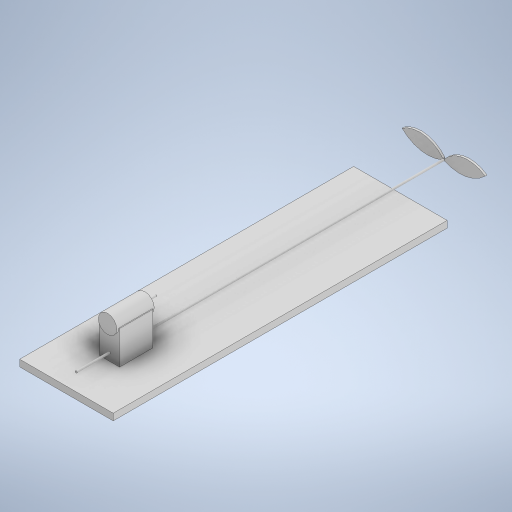
# Autodesk Inventor part: Motor Shaft
Saved by Autodesk Inventor 2024 (Build 280153000, 153)
## iProperties
Created: 2024-09-04
Part Number: Motor Shaft
Material: Generic
Document SubType Name: Modeling
Designer: srira
Density: 1 g/cm^3
Appearance: Default
Author: srira
Autodesk Inventor part; units mm, degrees
ref_plane "YZ Plane" through (0, 0, 0) normal (1, 0, 0) x (0, 1, 0)
ref_plane "XZ Plane" through (0, 0, 0) normal (0, 1, 0) x (-1, 0, 0)
ref_plane "XY Plane" through (0, 0, 0) normal (0, 0, 1) x (1, 0, 0)
sketch "Sketch1" plane through (0, 0, 0) normal (0, 1, 0) x (-1, 0, 0)
  line L0 (-70, 250) -> (70, 250)
  line L1 (70, 250) -> (70, -250)
  line L2 (70, -250) -> (-70, -250)
  line L3 (-70, -250) -> (-70, 250)
  line L4 (-70, 250) -> (70, -250) construction
  line L5 (70, 250) -> (-70, -250) construction
  point P0 (0, 0)
  dimension "d0" = 140
  dimension "d1" = 500
  constraints: 12 end point, 2 midpoint, 2 parallel, 1 horizontal, 1 perpendicular
  measures "d0" distance of L1.end L2.end
  measures "d1" distance of L0.end L1.end
extrude "Extrusion1" add sketch "Sketch1" along normal blind 10
sketch "Sketch2" plane through (0, 10, 0) normal (0, 1, 0) x (1, 0, 0)
  line L0 (15, -185.42) -> (-15, -185.42)
  line L1 (-15, -185.42) -> (-15, -135.42)
  line L2 (-15, -135.42) -> (15, -135.42)
  line L3 (15, -135.42) -> (15, -185.42)
  line L4 (15, -185.42) -> (-15, -135.42) construction
  line L5 (-15, -185.42) -> (15, -135.42) construction
  point P0 (0, 0)
  point P1 (0, -160.42)
  dimension "d4" = 30
  dimension "d5" = 50
  constraints: 12 end point, 2 midpoint, 2 parallel, 1 horizontal, 1 perpendicular
  measures "d4" distance of L1.end L2.end
  measures "d5" distance of L0.end L1.end
extrude "Extrusion2" add sketch "Sketch2" along normal blind 50
sketch "Sketch3" plane through (15, 10, 135.42) normal (0, 0, -1) x (-1, 0, 0)
  line L0 (30, 50) -> (0, 50) projected
  circle A0 centre (15, 50) radius 13.8
  point P0 (15, -10)
  point P1 (1.2, 50)
  point P2 (28.8, 50)
  dimension "d8" = 27.6
  constraints: 1 centre point, 1 midpoint
  measures "d8" diameter of A0
extrude "Extrusion3" cut sketch "Sketch3" against normal blind 50 contours A0 L0 picked at (18.5768, 45.8488)
sketch "Sketch4" plane through (-15, 10, 185.42) normal (0, 0, 1) x (1, 0, 0)
  circle A0 centre (15, 11.2668) radius 1.5
  point P0 (15, -10)
  dimension "d11" = 3
  constraints: 1 centre point
  measures "d11" diameter of A0
extrude "Extrusion5" add sketch "Sketch4" along normal blind 50 and the other way blind 500
sketch "Sketch5" plane through (0, 21.2668, -314.58) normal (0, 0, -1) x (-1, 0, 0)
  circle A0 centre (0, 0) radius 1.5 projected
  arc A1 (62.1392, 9.8676) -> (0, 0) centre (36.1239, -26.8945) ccw
  arc A2 (0, 0) -> (62.1392, 9.8676) centre (24.2766, 47.7112) ccw
  arc A3 (0, 0) -> (-62.1392, 9.8676) centre (-36.1239, -26.8945) ccw
  arc A4 (-62.1392, 9.8676) -> (0, 0) centre (-24.2766, 47.7112) ccw
  point P0 (0, -21.2668)
  point P1 (1.3463, -0.6614)
  point P2 (0.9157, 1.1881)
  point P3 (-1.3463, -0.6614)
  point P4 (-0.9157, 1.1881)
  constraints: 8 point on circle, 4 centre point, 2 other
extrude "Extrusion6" add sketch "Sketch5" along normal blind 3 contours A0 A1 A2 | A0 A4 A3 picked at (32.1855, 2.6766) picked at (-32.1855, 2.6766)
sketch "Sketch6" plane through (-15, 10, 185.42) normal (0, 0, 1) x (1, 0, 0)
  circle A0 centre (15, 50) radius 13.8
  point P0 (15, -10)
  dimension "d22" = 27.6
  constraints: 1 centre point
  measures "d22" diameter of A0
extrude "Extrusion7" add sketch "Sketch6" along normal blind 3 and the other way blind 53
sketch "Sketch7" plane through (0, 60, 132.42) normal (0, 0, -1) x (-1, 0, 0)
  circle A0 centre (0, 0) radius 1
  point P0 (0, -60)
  dimension "d27" = 2
  constraints: 1 centre point
  measures "d27" diameter of A0
extrude "Extrusion8" add sketch "Sketch7" along normal blind 17
body "Solid1"
